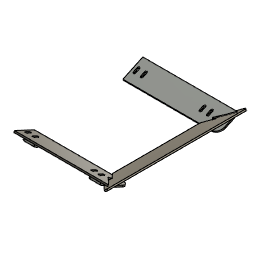
Led backlight edges (Autodesk Fusion 360 design; units mm, degrees)
Autodesk Fusion 360 part; units mm, degrees
note: some values were not read from the file. Set by a fixed rule: which sketch regions a step uses.
sketch "Sketch1" plane through (0, 0, 0) normal (0, 0, 1) x (1, 0, 0) in component "Holder"
  line L0 (118, -228) -> (118, -86)
  line L1 (118.5, -228.5) -> (118.5, -85.5)
  line L2 (10, -228) -> (10, -228.5)
  line L3 (10, -228) -> (10, -220)
  line L4 (10, -228.5) -> (118.5, -228.5)
  line L5 (5, -79) -> (5, -85.5)
  line L6 (15, -235) -> (15, -228.5)
  line L7 (105, -235) -> (115, -235)
  circle A0 centre (10, -232) radius 1.25
  line L8 (115, -235) -> (115, -228.5)
  line L9 (10, -220) -> (110, -220)
  line L10 (5, -85.5) -> (10, -85.5)
  line L11 (105, -79) -> (105, -85.5)
  line L12 (105, -235) -> (105, -228.5)
  line L13 (118.5, -85.5) -> (10, -85.5)
  line L14 (105, -79) -> (115, -79)
  line L15 (5, -228.5) -> (10, -228.5)
  line L16 (5, -235) -> (15, -235)
  line L17 (110, -94) -> (10, -94)
  line L18 (5, -235) -> (5, -228.5)
  circle A1 centre (10, -82) radius 1.25
  line L19 (10, -86) -> (10, -85.5)
  circle A2 centre (110, -82) radius 1.25
  line L20 (115, -79) -> (115, -85.5)
  line L21 (10, -94) -> (10, -86)
  line L22 (5, -79) -> (15, -79)
  line L23 (15, -79) -> (15, -85.5)
  line L24 (118, -86) -> (10, -86)
  line L25 (10, -228) -> (118, -228)
  circle A3 centre (110, -232) radius 1.25
  line L26 (110, -220) -> (110, -94)
  circle A4 centre (139, -235) radius 1.5
  line L27 (144, -231) -> (124, -231)
  line L28 (124, -239) -> (144, -239)
  line L29 (124, -239) -> (124, -231)
  line L30 (144, -239) -> (144, -231)
  line L31 (134, -239) -> (134, -231)
  line L32 (134, -239) -> (134.193, -239)
  point P0 (0, -220)
  dimension "d172" = 2.5
  dimension "d173" = 2.5
  dimension "d174" = 2.5
  dimension "d175" = 2.5
  dimension "d176" = 108
  dimension "d177" = 142
  dimension "d178" = 108.5
  dimension "d179" = 143
  dimension "d180" = 3
  constraint horizontal L14
  constraint horizontal L22
  constraint horizontal L16
  constraint horizontal L7
  constraint horizontal L25
  constraint vertical L0
  constraint horizontal L24
  constraint perpendicular L2 L25
  constraint horizontal L4
  constraint vertical L1
  constraint horizontal L13
  constraint coincident L8.end L4
  constraint perpendicular L4 L8
  constraint coincident L12.end L4
  constraint perpendicular L4 L12
  constraint coincident L6.end L4
  constraint perpendicular L4 L6
  constraint perpendicular L16 L18
  constraint coincident L11.end L13
  constraint perpendicular L11 L13
  constraint coincident L20.end L13
  constraint perpendicular L13 L20
  constraint perpendicular L13 L19
  constraint coincident L23.end L13
  constraint perpendicular L13 L23
  constraint perpendicular L5 L22
  constraint perpendicular L10 L19
  constraint perpendicular L3 L9
  constraint perpendicular L17 L21
  constraint horizontal L27
  constraint horizontal L28
  constraint perpendicular L27 L29
  constraint perpendicular L27 L30
  constraint midpoint L28 L31.start
  constraint midpoint L27 L31.end
  constraint coincident L28 L32.end
  constraint perpendicular L31 L32
  measures "d172" diameter of A3
  measures "d173" diameter of A0
  measures "d174" diameter of A1
  measures "d175" diameter of A2
  measures "d176" distance of L2.start L0.start
  measures "d177" distance of L2.start L19.start
  measures "d178" distance of L2.end L1.start
  measures "d179" distance of L2.end L10.end
  measures "d180" diameter of A4
extrude "Extrude1" add sketch "Sketch1" along normal blind 3 contours L27 L28 L30 L31 L32 makes body 1 in component "Holder"
sketch "Sketch4" plane through (144, 0, 0) normal (1, 0, 0) x (0, 1, 0) in component "Holder"
  line L0 (-231, 3) -> (-231, 5)
  line L1 (-231, 5) -> (-228.1, 5) construction
  line L2 (-231, 5) -> (-220.2775, 0)
  line L3 (-239, 0) -> (-231, 0)
  line L4 (-231, 0) -> (-231, 3)
  line L5 (-231, 3) -> (-239, 3)
  line L6 (-239, 3) -> (-239, 0)
  line L7 (-231, 5) -> (-240.0631, 9.2262)
  line L8 (-231, 5) -> (-221, 5) construction
  line L9 (-240.0631, 9.2262) -> (-236.6821, 16.4766)
  line L10 (-231, 5) -> (-227.619, 12.2505)
  line L11 (-227.619, 12.2505) -> (-236.6821, 16.4766)
  dimension "d187" = 155
  dimension "d188" = 10
  dimension "d189" = 8
  dimension "d190" = 8
  constraint horizontal L1
  constraint horizontal L8
  constraint parallel L2 L7
  constraint perpendicular L7 L9
  constraint perpendicular L7 L10
  measures "d187" angle of L7 L8
  measures "d188" distance of L0.end L7.end
  measures "d189" distance of L7.end L9.end
  measures "d190" distance of L0.end L10.end
extrude "Extrude2" add sketch "Sketch1" along normal blind 9 contours L27 L28 L29 L31 bodies 1 in component "Holder"
extrude "Extrude3" cut sketch "Sketch4" against normal blind 23 contours L7 L9 L10 L11 bodies 1 in component "Holder"
sketch "Sketch2" plane through (0, -39.3429, -84.3712) normal (0, 0.422618, 0.906308) x (-1, 0, 0) in component "Holder"
  line L0 (-124, 211.4702) -> (-124, 220.2972)
  line L1 (-124, 220.2972) -> (-134, 220.2972)
  line L2 (-134, 220.2972) -> (-134, 211.4702)
  line L3 (-134, 211.4702) -> (-124, 211.4702)
  circle A0 centre (-129, 214.8837) radius 1.35
  dimension "d198" = 2.7
  measures "d198" diameter of A0
extrude "Extrude5" cut sketch "Sketch2" against normal blind 8 contours A0 bodies 1 in component "Holder"
fillet "Fillet1" radius 3 4 edges at (144, -239, 1.5) (144, -231, 1.5) (124, -239, 4.3652) (124, -231, 2.5) on bodies 1 in component "Holder"
fillet "Fillet2" radius 3 2 edges at (134, -239, 5.8652) (134, -231, 4) on bodies 1 in component "Holder"
mirror "MirrorComponent5" about plane through (0, 0, 0) normal (0, 0, 1) of bodies 1 makes body 2 in component "Holder(Mirror)"
sketch "Sketch1 (2)" plane through (0, 0, 0) normal (0, 0, 1) x (1, 0, 0) in component "SidePanel"
  line L0 (34, -235) -> (34, -213)
  arc A0 (140.5, -225) -> (137.5, -225) centre (139, -225) ccw
  line L1 (137.5, -225) -> (137.5, -231)
  line L2 (140.5, -225) -> (140.5, -231)
  arc A1 (137.5, -231) -> (140.5, -231) centre (139, -231) ccw
  line L3 (130.5, -225) -> (130.5, -231)
  arc A2 (130.5, -225) -> (127.5, -225) centre (129, -225) ccw
  line L4 (127.5, -225) -> (127.5, -231)
  arc A3 (127.5, -231) -> (130.5, -231) centre (129, -231) ccw
  arc A4 (40.5, -225) -> (37.5, -225) centre (39, -225) ccw
  line L5 (37.5, -225) -> (37.5, -231)
  line L6 (40.5, -225) -> (40.5, -231)
  arc A5 (37.5, -231) -> (40.5, -231) centre (39, -231) ccw
  line L7 (50.5, -225) -> (50.5, -231)
  line L8 (47.5, -225) -> (47.5, -231)
  arc A6 (50.5, -225) -> (47.5, -225) centre (49, -225) ccw
  arc A7 (47.5, -231) -> (50.5, -231) centre (49, -231) ccw
  line L9 (145.1924, -225.0208) -> (155.1716, -235)
  line L10 (148.7279, -221.4853) -> (145.1924, -225.0208)
  arc A8 (164, -223) -> (154, -213) centre (154, -223) ccw
  line L11 (154, -213) -> (34, -213)
  line L12 (164, -223) -> (164, -233)
  line L13 (161.2727, -234.03) -> (148.7279, -221.4853)
  line L14 (34, -235) -> (34, -243)
  line L15 (161.2727, -234.03) -> (164, -237.1258)
  line L16 (155.1716, -235) -> (162.2195, -243)
  line L17 (164, -233) -> (164, -237.1258)
  line L18 (162.2195, -243) -> (34, -243)
  dimension "d205" = 22
  dimension "d256" = 5
  constraint tangent A0 L1
  constraint vertical L1
  constraint tangent A0 L2
  constraint vertical L2
  constraint tangent L2 A1
  constraint tangent L1 A1
  constraint tangent A2 L4
  constraint vertical L4
  constraint tangent L3 A2
  constraint vertical L3
  constraint tangent L3 A3
  constraint tangent L4 A3
  constraint tangent A4 L5
  constraint vertical L5
  constraint tangent A4 L6
  constraint vertical L6
  constraint tangent L6 A5
  constraint tangent L5 A5
  constraint tangent L8 A6
  constraint vertical L8
  constraint tangent L7 A6
  constraint vertical L7
  constraint tangent L7 A7
  constraint tangent L8 A7
  constraint tangent A8 L12
  constraint vertical L12
  constraint perpendicular L10 L13
  constraint parallel L15 L16
  constraint parallel L12 L17
  constraint perpendicular L14 L18
  measures "d205" distance of L0.start L0.end
  measures "d256" distance of L9.start L10.start
extrude "Extrude1'" add sketch "Sketch1 (2)" along normal blind 2 separate body makes body 3 in component "SidePanel"
sketch "Sketch1 (3)" plane through (0, 0, 0) normal (0, 0, 1) x (1, 0, 0) in component "BackPanel"
  line L0 (170, -220) -> (170, -100)
  line L1 (200, -220) -> (200, -221)
  line L2 (200, -221) -> (200, -247.2727)
  line L3 (180.9009, -229.9099) -> (180.9009, -240.9099)
  line L4 (180.9009, -240.9099) -> (197.1796, -255.7087)
  line L5 (200, -247.2727) -> (200, -254.2727)
  arc A0 (197.1796, -255.7087) -> (200, -254.2727) centre (198.2242, -254.2727) ccw
  line L6 (170, -220) -> (180.9009, -229.9099)
  line L7 (180.9009, -90) -> (180.9009, -79)
  line L8 (180.9009, -79) -> (197.1796, -64.2012)
  line L9 (200, -98.9099) -> (200, -72.6372)
  line L10 (200, -72.6372) -> (200, -65.6372)
  arc A1 (197.1796, -64.2012) -> (200, -65.6372) centre (198.2242, -65.6372) cw
  line L11 (200, -98.9099) -> (200, -220)
  line L12 (180.9009, -90) -> (170, -100)
  dimension "d215" = 120
  dimension "d258" = 11
  dimension "d260" = 22
  dimension "d261" = 7
  dimension "d262" = 11
  dimension "d264" = 7
  constraint vertical L0
  constraint parallel L2 L5
  constraint tangent L5 A0
  constraint parallel L9 L10
  constraint tangent L10 A1
  constraint parallel L1 L11
  measures "d215" distance of L0.start L0.end
  measures "d258" distance of L3.start L3.end
  measures "d260" distance of L3.end L4.end
  measures "d261" distance of L2.end L5.end
  measures "d262" distance of L7.end L7.start
  measures "d264" distance of L9.end L10.end
extrude "Extrude1''" add sketch "Sketch1 (3)" along normal blind 2 separate body makes body 4 in component "BackPanel"
component "Holder" placed x (1, 0, 0) y (0, 1, 0) z (0, 0, 1) at (0, 0, 0)
component "SidePanel" placed x (1, 0, 0) y (0, 0.906308, -0.422618) z (0, 0.422618, 0.906308) at (0, -29.7449, -88.6171)
component "Holder(Mirror)" placed x (-1, 0, 0) y (0, 1, 0) z (0, 0, -1) at (178, 0, 0)
component "Holder" placed x (-1, 0, 0) y (0, -1, 0) z (0, 0, 1) at (178.0112, -320.5376, 0)
component "Holder(Mirror)" placed x (1, 0, 0) y (0, -1, 0) z (0, 0, -1) at (0.0112, -320.5376, 0)
component "SidePanel" placed x (1, 0, 0) y (0, -0.906308, -0.422618) z (0, 0.422618, -0.906308) at (0, -294.2917, -87.4665)
component "BackPanel" placed x (0.906308, 0, 0.422618) y (0, 1, 0) z (-0.422618, 0, 0.906308) at (-13.9211, -1, -70.0166)
equation "d187 = 180 deg - 25 deg"
